Autodesk Fusion 360 part; units mm, degrees
(part 5 of 14)
  line L2013 (32.35, 52.7992) -> (32.35, 53.4088)
  line L2014 (32.35, 51.5292) -> (32.35, 52.1388)
  line L2015 (32.983, 52.1388) -> (32.733, 52.1388)
  line L2016 (56.818, 14.4648) -> (56.818, 13.8552)
  line L2017 (33.366, 53.4088) -> (33.366, 52.7992)
  line L2018 (32.733, 52.7992) -> (32.983, 52.7992)
  line L2019 (57.9882, 55.626) -> (58.5978, 55.626)
  line L2020 (33.408, 52.134) -> (32.308, 52.134)
  line L2021 (33.366, 53.4088) -> (33.366, 52.7992)
  line L2022 (27.259, 50.123) -> (27.859, 50.123)
  line L2023 (27.8638, 50.165) -> (27.2542, 50.165)
  line L2024 (27.259, 51.223) -> (27.259, 50.123)
  line L2025 (32.308, 52.134) -> (32.308, 51.534)
  line L2026 (58.5978, 54.993) -> (58.5978, 55.243)
  line L2027 (21.209, 34.3408) -> (21.209, 33.7312)
  line L2028 (56.86, 14.46) -> (55.76, 14.46)
  line L2029 (34.76, 35.491) -> (34.76, 34.891)
  line L2030 (32.308, 53.404) -> (32.308, 52.804)
  line L2031 (27.2542, 50.548) -> (27.8638, 50.548)
  line L2032 (27.859, 50.123) -> (27.859, 51.223)
  line L2033 (32.308, 52.804) -> (33.408, 52.804)
  line L2034 (33.366, 52.1388) -> (33.366, 51.5292)
  line L2035 (20.826, 33.7312) -> (20.826, 34.3408)
  line L2036 (20.193, 34.3408) -> (21.209, 34.3408)
  line L2037 (27.8638, 51.181) -> (27.8638, 50.165)
  line L2038 (32.35, 52.7992) -> (32.35, 53.4088)
  line L2039 (20.193, 34.3408) -> (21.209, 34.3408)
  line L2040 (27.2542, 50.165) -> (27.2542, 51.181)
  line L2041 (33.408, 51.534) -> (33.408, 52.134)
  line L2042 (27.8638, 51.181) -> (27.8638, 50.165)
  line L2043 (55.76, 14.46) -> (55.76, 13.86)
  line L2044 (56.435, 14.4648) -> (56.185, 14.4648)
  line L2045 (40.5638, 44.958) -> (40.5638, 43.942)
  line L2046 (39.9542, 44.958) -> (40.5638, 44.958)
  line L2047 (35.435, 36.7658) -> (35.185, 36.7658)
  line L2048 (34.802, 34.8862) -> (34.802, 35.4958)
  line L2049 (41.7068, 44.958) -> (41.7068, 43.942)
  line L2050 (35.818, 36.7658) -> (35.818, 36.1562)
  line L2051 (57.9882, 54.61) -> (57.9882, 55.626)
  line L2052 (35.818, 36.1562) -> (34.802, 36.1562)
  line L2053 (39.9542, 44.325) -> (40.5638, 44.325)
  line L2054 (39.9542, 44.958) -> (40.5638, 44.958)
  line L2055 (35.818, 35.4958) -> (35.818, 34.8862)
  line L2056 (41.102, 43.9) -> (41.702, 43.9)
  line L2057 (58.5978, 55.243) -> (57.9882, 55.243)
  line L2058 (35.185, 36.1562) -> (35.435, 36.1562)
  line L2059 (57.9882, 54.61) -> (57.9882, 55.626)
  line L2060 (27.8638, 50.548) -> (27.8638, 50.798)
  line L2061 (39.959, 45) -> (39.959, 43.9)
  line L2062 (35.185, 36.7658) -> (35.185, 36.1562)
  line L2063 (55.802, 14.4648) -> (56.818, 14.4648)
  line L2064 (34.802, 35.4958) -> (35.818, 35.4958)
  line L2065 (35.86, 35.491) -> (34.76, 35.491)
  line L2066 (58.5978, 55.626) -> (58.5978, 54.61)
  line L2067 (34.76, 34.891) -> (35.86, 34.891)
  line L2068 (27.2542, 50.798) -> (27.2542, 50.548)
  line L2069 (35.435, 35.4958) -> (35.185, 35.4958)
  line L2070 (39.9542, 43.942) -> (39.9542, 44.958)
  line L2071 (56.818, 13.8552) -> (55.802, 13.8552)
  line L2072 (41.0972, 44.958) -> (41.7068, 44.958)
  line L2073 (41.702, 43.9) -> (41.702, 45)
  line L2074 (55.76, 13.86) -> (56.86, 13.86)
  line L2075 (35.185, 35.4958) -> (35.185, 34.8862)
  line L2076 (56.185, 14.4648) -> (56.185, 13.8552)
  line L2077 (27.2542, 50.165) -> (27.2542, 51.181)
  line L2078 (35.86, 36.761) -> (34.76, 36.761)
  line L2079 (34.802, 35.4958) -> (35.818, 35.4958)
  line L2080 (41.7068, 43.942) -> (41.0972, 43.942)
  line L2081 (35.86, 36.161) -> (35.86, 36.761)
  line L2082 (56.435, 13.8552) -> (56.435, 14.4648)
  line L2083 (57.9882, 54.993) -> (58.5978, 54.993)
  line L2084 (41.7068, 43.942) -> (41.0972, 43.942)
  line L2085 (41.702, 45) -> (41.102, 45)
  line L2086 (55.802, 14.4648) -> (56.818, 14.4648)
  line L2087 (58.593, 55.668) -> (57.993, 55.668)
  line L2088 (41.0972, 44.325) -> (41.7068, 44.325)
  line L2089 (35.185, 34.8862) -> (35.435, 34.8862)
  line L2090 (39.959, 43.9) -> (40.559, 43.9)
  line L2091 (39.9542, 43.942) -> (39.9542, 44.958)
  line L2092 (55.802, 13.8552) -> (55.802, 14.4648)
  line L2093 (40.5638, 43.942) -> (39.9542, 43.942)
  line L2094 (58.593, 54.568) -> (58.593, 55.668)
  line L2095 (34.802, 34.8862) -> (34.802, 35.4958)
  line L2096 (58.5978, 54.61) -> (57.9882, 54.61)
  line L2097 (40.5638, 44.958) -> (40.5638, 43.942)
  line L2098 (57.9882, 55.243) -> (57.9882, 54.993)
  line L2099 (27.8638, 50.165) -> (27.2542, 50.165)
  line L2100 (34.802, 36.7658) -> (35.818, 36.7658)
  line L2101 (35.818, 34.8862) -> (34.802, 34.8862)
  line L2102 (35.86, 34.891) -> (35.86, 35.491)
  line L2103 (27.8638, 50.798) -> (27.2542, 50.798)
  line L2104 (40.5638, 43.942) -> (39.9542, 43.942)
  line L2105 (34.76, 36.161) -> (35.86, 36.161)
  line L2106 (41.7068, 44.575) -> (41.0972, 44.575)
  line L2107 (57.993, 55.668) -> (57.993, 54.568)
  line L2108 (41.0972, 43.942) -> (41.0972, 44.958)
  line L2109 (34.802, 31.3302) -> (34.802, 31.9398)
  line L2110 (35.185, 31.3302) -> (35.435, 31.3302)
  line L2111 (41.0972, 44.575) -> (41.0972, 44.325)
  line L2112 (35.435, 31.3302) -> (35.435, 31.9398)
  line L2113 (35.86, 31.935) -> (34.76, 31.935)
  line L2114 (37.6682, 43.942) -> (37.6682, 44.958)
  line L2115 (34.802, 31.9398) -> (35.818, 31.9398)
  line L2116 (38.816, 45) -> (38.816, 43.9)
  line L2117 (35.818, 31.9398) -> (35.818, 31.3302)
  line L2118 (34.802, 36.1562) -> (34.802, 36.7658)
  line L2119 (38.2778, 44.575) -> (37.6682, 44.575)
  line L2120 (41.102, 45) -> (41.102, 43.9)
  line L2121 (34.76, 31.935) -> (34.76, 31.335)
  line L2122 (39.4208, 43.942) -> (38.8112, 43.942)
  line L2123 (38.273, 45) -> (37.673, 45)
  line L2124 (38.2778, 43.942) -> (37.6682, 43.942)
  line L2125 (39.4208, 44.958) -> (39.4208, 43.942)
  line L2126 (37.673, 43.9) -> (38.273, 43.9)
  line L2127 (38.816, 43.9) -> (39.416, 43.9)
  line L2128 (38.8112, 43.942) -> (38.8112, 44.958)
  line L2129 (34.76, 36.761) -> (34.76, 36.161)
  line L2130 (38.2778, 44.958) -> (38.2778, 43.942)
  line L2131 (38.8112, 43.942) -> (38.8112, 44.958)
  line L2132 (41.7068, 44.958) -> (41.7068, 43.942)
  line L2133 (39.416, 43.9) -> (39.416, 45)
  line L2134 (35.818, 31.9398) -> (35.818, 31.3302)
  line L2135 (35.435, 31.9398) -> (35.185, 31.9398)
  line L2136 (37.6682, 44.958) -> (38.2778, 44.958)
  line L2137 (38.2778, 43.942) -> (37.6682, 43.942)
  line L2138 (38.273, 43.9) -> (38.273, 45)
  line L2139 (35.86, 31.335) -> (35.86, 31.935)
  line L2140 (35.185, 31.9398) -> (35.185, 31.3302)
  line L2141 (38.2778, 44.325) -> (38.2778, 44.575)
  line L2142 (38.2778, 44.958) -> (38.2778, 43.942)
  line L2143 (34.802, 31.3302) -> (34.802, 31.9398)
  line L2144 (35.818, 31.3302) -> (34.802, 31.3302)
  line L2145 (39.4208, 44.575) -> (38.8112, 44.575)
  line L2146 (39.4208, 44.325) -> (39.4208, 44.575)
  line L2147 (35.818, 36.7658) -> (35.818, 36.1562)
  line L2148 (37.6682, 44.325) -> (38.2778, 44.325)
  line L2149 (35.435, 36.1562) -> (35.435, 36.7658)
  line L2150 (37.6682, 44.958) -> (38.2778, 44.958)
  line L2151 (40.5638, 44.325) -> (40.5638, 44.575)
  line L2152 (38.8112, 44.958) -> (39.4208, 44.958)
  line L2153 (41.0972, 44.958) -> (41.7068, 44.958)
  line L2154 (37.6682, 44.575) -> (37.6682, 44.325)
  line L2155 (40.5638, 44.575) -> (39.9542, 44.575)
  line L2156 (40.559, 43.9) -> (40.559, 45)
  line L2157 (39.4208, 44.958) -> (39.4208, 43.942)
  line L2158 (38.8112, 44.575) -> (38.8112, 44.325)
  line L2159 (34.76, 31.335) -> (35.86, 31.335)
  line L2160 (40.559, 45) -> (39.959, 45)
  line L2161 (37.673, 45) -> (37.673, 43.9)
  line L2162 (34.802, 36.7658) -> (35.818, 36.7658)
  line L2163 (41.0972, 43.942) -> (41.0972, 44.958)
  line L2164 (41.7068, 44.325) -> (41.7068, 44.575)
  line L2165 (39.9542, 44.575) -> (39.9542, 44.325)
  line L2166 (34.802, 36.1562) -> (34.802, 36.7658)
  line L2167 (37.6682, 43.942) -> (37.6682, 44.958)
  line L2168 (39.416, 45) -> (38.816, 45)
  line L2169 (35.818, 36.1562) -> (34.802, 36.1562)
  line L2170 (35.818, 31.3302) -> (34.802, 31.3302)
  line L2171 (38.8112, 44.958) -> (39.4208, 44.958)
  line L2172 (39.4208, 43.942) -> (38.8112, 43.942)
  line L2173 (34.802, 32.4732) -> (34.802, 33.0828)
  line L2174 (34.685, 28.162) -> (34.685, 27.562)
  line L2175 (35.36, 27.5572) -> (35.36, 28.1668)
  line L2176 (35.435, 33.0828) -> (35.185, 33.0828)
  line L2177 (35.818, 33.0828) -> (35.818, 32.4732)
  line L2178 (35.818, 32.4732) -> (34.802, 32.4732)
  line L2179 (36.5252, 44.325) -> (37.1348, 44.325)
  line L2180 (35.743, 27.5572) -> (34.727, 27.5572)
  line L2181 (37.1348, 44.958) -> (37.1348, 43.942)
  line L2182 (76.4032, 61.214) -> (76.4032, 62.23)
  line L2183 (35.818, 32.4732) -> (34.802, 32.4732)
  line L2184 (36.53, 43.9) -> (37.13, 43.9)
  line L2185 (37.13, 43.9) -> (37.13, 45)
  line L2186 (37.1348, 44.958) -> (37.1348, 43.942)
  line L2187 (34.802, 31.9398) -> (35.818, 31.9398)
  line L2188 (34.727, 27.5572) -> (34.727, 28.1668)
  line L2189 (34.802, 33.0828) -> (35.818, 33.0828)
  line L2190 (35.743, 30.4528) -> (35.743, 29.8432)
  line L2191 (35.785, 28.705) -> (35.785, 29.305)
  line L2192 (36.5252, 44.958) -> (37.1348, 44.958)
  line L2193 (34.76, 33.078) -> (34.76, 32.478)
  line L2194 (35.743, 28.1668) -> (35.743, 27.5572)
  line L2195 (35.818, 33.0828) -> (35.818, 32.4732)
  line L2196 (35.785, 29.305) -> (34.685, 29.305)
  line L2197 (35.185, 33.0828) -> (35.185, 32.4732)
  line L2198 (35.11, 27.5572) -> (35.36, 27.5572)
  line L2199 (34.727, 28.7002) -> (34.727, 29.3098)
  line L2200 (34.802, 32.4732) -> (34.802, 33.0828)
  line L2201 (35.11, 30.4528) -> (35.11, 29.8432)
  line L2202 (35.743, 28.7002) -> (34.727, 28.7002)
  line L2203 (35.86, 32.478) -> (35.86, 33.078)
  line L2204 (35.743, 28.7002) -> (34.727, 28.7002)
  line L2205 (35.36, 28.1668) -> (35.11, 28.1668)
  line L2206 (34.727, 29.3098) -> (35.743, 29.3098)
  line L2207 (34.727, 28.7002) -> (34.727, 29.3098)
  line L2208 (35.785, 29.848) -> (35.785, 30.448)
  line L2209 (76.408, 62.272) -> (76.408, 61.172)
  line L2210 (34.685, 27.562) -> (35.785, 27.562)
  line L2211 (35.185, 32.4732) -> (35.435, 32.4732)
  line L2212 (35.11, 29.8432) -> (35.36, 29.8432)
  line L2213 (36.53, 45) -> (36.53, 43.9)
  line L2214 (35.36, 29.3098) -> (35.11, 29.3098)
  line L2215 (34.727, 28.1668) -> (35.743, 28.1668)
  line L2216 (35.11, 29.3098) -> (35.11, 28.7002)
  line L2217 (35.11, 28.1668) -> (35.11, 27.5572)
  line L2218 (34.685, 28.705) -> (35.785, 28.705)
  line L2219 (34.685, 29.305) -> (34.685, 28.705)
  line L2220 (35.785, 27.562) -> (35.785, 28.162)
  line L2221 (34.727, 28.1668) -> (35.743, 28.1668)
  line L2222 (34.727, 29.3098) -> (35.743, 29.3098)
  line L2223 (34.76, 32.478) -> (35.86, 32.478)
  line L2224 (35.435, 32.4732) -> (35.435, 33.0828)
  line L2225 (35.36, 28.7002) -> (35.36, 29.3098)
  line L2226 (38.8112, 44.325) -> (39.4208, 44.325)
  line L2227 (34.727, 27.5572) -> (34.727, 28.1668)
  line L2228 (35.743, 29.3098) -> (35.743, 28.7002)
  line L2229 (35.743, 28.1668) -> (35.743, 27.5572)
  line L2230 (35.86, 33.078) -> (34.76, 33.078)
  line L2231 (35.743, 27.5572) -> (34.727, 27.5572)
  line L2232 (34.802, 33.0828) -> (35.818, 33.0828)
  line L2233 (37.13, 45) -> (36.53, 45)
  line L2234 (35.785, 28.162) -> (34.685, 28.162)
  line L2235 (35.11, 28.7002) -> (35.36, 28.7002)
  line L2236 (35.743, 29.3098) -> (35.743, 28.7002)
  line L2237 (51.6128, 43.688) -> (51.0032, 43.688)
  line L2238 (37.1348, 43.942) -> (36.5252, 43.942)
  line L2239 (52.7304, 58.6438) -> (52.4764, 58.1358)
  line L2240 (51.608, 43.646) -> (51.608, 44.746)
  line L2241 (51.0032, 43.688) -> (51.0032, 44.704)
  line L2242 (51.0032, 44.704) -> (51.6128, 44.704)
  line L2243 (35.743, 29.8432) -> (34.727, 29.8432)
  line L2244 (55.4736, 60.9092) -> (54.5084, 60.9092)
  line L2245 (54.5084, 60.9092) -> (54.5084, 59.2328)
  line L2246 (55.4736, 59.2328) -> (55.4736, 60.9092)
  line L2247 (37.1348, 43.942) -> (36.5252, 43.942)
  line L2248 (52.9336, 59.2328) -> (52.9336, 60.9092)
  line L2249 (54.5084, 60.9092) -> (54.5084, 59.2328)
  line L2250 (51.6128, 44.071) -> (51.6128, 44.321)
  line L2251 (35.743, 30.4528) -> (35.743, 29.8432)
  line L2252 (36.5252, 44.958) -> (37.1348, 44.958)
  line L2253 (77.0128, 61.214) -> (76.4032, 61.214)
  line L2254 (77.008, 62.272) -> (76.408, 62.272)
  line L2255 (54.511, 60.946) -> (54.511, 59.196)
  line L2256 (52.4764, 58.1358) -> (52.2224, 58.6438)
  line L2257 (36.5252, 43.942) -> (36.5252, 44.958)
  line L2258 (34.727, 30.4528) -> (35.743, 30.4528)
  line L2259 (52.901, 60.771) -> (52.001, 60.771)
  line L2260 (52.2224, 58.6438) -> (52.7304, 58.6438)
  line L2261 (51.9684, 60.9092) -> (51.9684, 59.2328)
  line L2262 (52.9336, 60.9092) -> (51.9684, 60.9092)
  line L2263 (55.4736, 59.2328) -> (55.4736, 60.9092)
  line L2264 (54.5084, 59.2328) -> (55.4736, 59.2328)
  arc A1277 (52.2224, 58.085) -> (52.2224, 58.1866) centre (52.2224, 58.1358) ccw
  line L2265 (35.785, 30.448) -> (34.685, 30.448)
  arc A1278 (52.4764, 58.1866) -> (52.4764, 58.085) centre (52.4764, 58.1358) ccw
  line L2266 (51.008, 44.746) -> (51.008, 43.646)
  line L2267 (77.0128, 62.23) -> (77.0128, 61.214)
  line L2268 (34.685, 29.848) -> (35.785, 29.848)
  line L2269 (34.727, 29.8432) -> (34.727, 30.4528)
  line L2270 (37.1348, 44.575) -> (36.5252, 44.575)
  line L2271 (76.4032, 61.847) -> (76.4032, 61.597)
  line L2272 (51.0032, 43.688) -> (51.0032, 44.704)
  line L2273 (51.6128, 43.688) -> (51.0032, 43.688)
  line L2274 (76.4032, 62.23) -> (77.0128, 62.23)
  line L2275 (77.0128, 61.597) -> (77.0128, 61.847)
  line L2276 (51.6128, 44.704) -> (51.6128, 43.688)
  line L2277 (52.9336, 60.9092) -> (51.9684, 60.9092)
  line L2278 (77.0128, 61.847) -> (76.4032, 61.847)
  line L2279 (34.727, 30.4528) -> (35.743, 30.4528)
  line L2280 (35.36, 30.4528) -> (35.11, 30.4528)
  line L2281 (51.008, 43.646) -> (51.608, 43.646)
  line L2282 (77.008, 61.172) -> (77.008, 62.272)
  line L2283 (77.0128, 61.214) -> (76.4032, 61.214)
  line L2284 (51.608, 44.746) -> (51.008, 44.746)
  line L2285 (34.685, 30.448) -> (34.685, 29.848)
  line L2286 (51.6128, 44.321) -> (51.0032, 44.321)
  line L2287 (76.408, 61.172) -> (77.008, 61.172)
  line L2288 (36.5252, 44.575) -> (36.5252, 44.325)
  line L2289 (36.5252, 43.942) -> (36.5252, 44.958)
  line L2290 (35.36, 29.8432) -> (35.36, 30.4528)
  line L2291 (76.4032, 62.23) -> (77.0128, 62.23)
  line L2292 (37.1348, 44.325) -> (37.1348, 44.575)
  line L2293 (34.727, 29.8432) -> (34.727, 30.4528)
  line L2294 (35.743, 29.8432) -> (34.727, 29.8432)
  line L2295 (76.4032, 61.214) -> (76.4032, 62.23)
  line L2296 (54.5084, 59.2328) -> (55.4736, 59.2328)
  line L2297 (77.0128, 62.23) -> (77.0128, 61.214)
  line L2298 (76.4032, 61.597) -> (77.0128, 61.597)
  line L2299 (58.0136, 59.2328) -> (58.0136, 60.9092)
  arc A1279 (54.7624, 58.6946) -> (54.7624, 58.593) centre (54.7624, 58.6438) ccw
  line L2300 (52.9336, 59.2328) -> (52.9336, 60.9092)
  arc A1280 (57.3024, 58.085) -> (57.3024, 58.1866) centre (57.3024, 58.1358) ccw
  line L2301 (57.981, 60.771) -> (57.081, 60.771)
  arc A1281 (57.3024, 58.593) -> (57.3024, 58.6946) centre (57.3024, 58.6438) ccw
  arc A1282 (54.7624, 58.593) -> (54.7624, 58.6946) centre (54.7624, 58.6438) ccw
  line L2302 (51.971, 60.946) -> (51.971, 59.196)
  line L2303 (57.981, 60.771) -> (57.081, 60.771)
  line L2304 (52.931, 60.946) -> (51.971, 60.946)
  line L2305 (58.0136, 60.9092) -> (57.0484, 60.9092)
  line L2306 (51.0032, 44.704) -> (51.6128, 44.704)
  arc A1283 (52.7304, 58.1866) -> (52.7304, 58.085) centre (52.7304, 58.1358) ccw
  arc A1284 (57.8104, 58.593) -> (57.8104, 58.6946) centre (57.8104, 58.6438) ccw
  line L2307 (57.8104, 58.6438) -> (57.5564, 58.1358)
  line L2308 (58.0136, 60.9092) -> (57.0484, 60.9092)
  line L2309 (51.0032, 44.321) -> (51.0032, 44.071)
  arc A1285 (55.2704, 58.1866) -> (55.2704, 58.085) centre (55.2704, 58.1358) ccw
  line L2310 (58.011, 59.196) -> (58.011, 60.946)
  line L2311 (51.9684, 59.2328) -> (52.9336, 59.2328)
  arc A1286 (52.7304, 58.085) -> (52.7304, 58.1866) centre (52.7304, 58.1358) ccw
  line L2312 (52.7304, 58.1358) -> (52.2224, 58.1358)
  arc A1287 (55.2704, 58.6946) -> (55.2704, 58.593) centre (55.2704, 58.6438) ccw
  arc A1288 (52.2224, 58.6946) -> (52.2224, 58.593) centre (52.2224, 58.6438) ccw
  line L2313 (57.5564, 58.1358) -> (57.3024, 58.6438)
  arc A1289 (55.2704, 58.593) -> (55.2704, 58.6946) centre (55.2704, 58.6438) ccw
  arc A1290 (55.0164, 58.085) -> (55.0164, 58.1866) centre (55.0164, 58.1358) ccw
  arc A1291 (55.0164, 58.1866) -> (55.0164, 58.085) centre (55.0164, 58.1358) ccw
  arc A1292 (57.5564, 58.085) -> (57.5564, 58.1866) centre (57.5564, 58.1358) ccw
  arc A1293 (57.3024, 58.6946) -> (57.3024, 58.593) centre (57.3024, 58.6438) ccw
  line L2314 (55.441, 60.771) -> (54.541, 60.771)
  arc A1294 (57.3024, 58.1866) -> (57.3024, 58.085) centre (57.3024, 58.1358) ccw
  arc A1295 (52.4764, 58.085) -> (52.4764, 58.1866) centre (52.4764, 58.1358) ccw
  line L2315 (57.3024, 58.6438) -> (57.8104, 58.6438)
  line L2316 (57.051, 60.946) -> (57.051, 59.196)
  arc A1296 (57.5564, 58.1866) -> (57.5564, 58.085) centre (57.5564, 58.1358) ccw
  arc A1297 (57.8104, 58.1866) -> (57.8104, 58.085) centre (57.8104, 58.1358) ccw
  arc A1298 (52.2224, 58.1866) -> (52.2224, 58.085) centre (52.2224, 58.1358) ccw
  line L2317 (54.511, 59.196) -> (55.471, 59.196)
  line L2318 (57.0484, 60.9092) -> (57.0484, 59.2328)
  line L2319 (52.901, 59.371) -> (52.001, 59.371)
  arc A1299 (57.8104, 58.085) -> (57.8104, 58.1866) centre (57.8104, 58.1358) ccw
  line L2320 (52.931, 59.196) -> (52.931, 60.946)
  line L2321 (55.4736, 60.9092) -> (54.5084, 60.9092)
  line L2322 (52.901, 59.371) -> (52.001, 59.371)
  line L2323 (55.441, 59.371) -> (54.541, 59.371)
  line L2324 (51.0032, 44.071) -> (51.6128, 44.071)
  arc A1300 (52.2224, 58.593) -> (52.2224, 58.6946) centre (52.2224, 58.6438) ccw
  line L2325 (57.0484, 60.9092) -> (57.0484, 59.2328)
  arc A1301 (57.8104, 58.6946) -> (57.8104, 58.593) centre (57.8104, 58.6438) ccw
  arc A1302 (54.7624, 58.085) -> (54.7624, 58.1866) centre (54.7624, 58.1358) ccw
  line L2326 (52.901, 59.371) -> (52.001, 59.371)
  line L2327 (51.6128, 44.704) -> (51.6128, 43.688)
  line L2328 (55.471, 59.196) -> (55.471, 60.946)
  line L2329 (52.901, 60.771) -> (52.001, 60.771)
  line L2330 (51.9684, 59.2328) -> (52.9336, 59.2328)
  line L2331 (51.9684, 60.9092) -> (51.9684, 59.2328)
  arc A1303 (52.7304, 58.593) -> (52.7304, 58.6946) centre (52.7304, 58.6438) ccw
  arc A1304 (52.7304, 58.6946) -> (52.7304, 58.593) centre (52.7304, 58.6438) ccw
  line L2332 (55.471, 60.946) -> (54.511, 60.946)
  line L2333 (52.901, 60.771) -> (52.001, 60.771)
  line L2334 (51.971, 59.196) -> (52.931, 59.196)
  line L2335 (55.441, 60.771) -> (54.541, 60.771)
  line L2336 (58.0136, 59.2328) -> (58.0136, 60.9092)
  line L2337 (27.559, 10.5918) -> (27.559, 12.0142)
  line L2338 (25.566, 10.628) -> (25.566, 11.978)
  line L2339 (25.273, 12.0142) -> (25.273, 10.5918)
  line L2340 (15.41, 25.437) -> (17.61, 25.437)
  arc A1305 (55.2704, 58.085) -> (55.2704, 58.1866) centre (55.2704, 58.1358) ccw
  line L2341 (11.684, 23.3172) -> (11.684, 21.8948)
  line L2342 (28.575, 24.3078) -> (28.575, 25.7302)
  line L2343 (58.011, 60.946) -> (57.051, 60.946)
  line L2344 (57.8104, 58.1358) -> (57.3024, 58.1358)
  line L2345 (17.61, 26.887) -> (15.41, 26.887)
  line L2346 (13.97, 21.8948) -> (13.97, 23.3172)
  line L2347 (11.727, 23.331) -> (11.727, 21.881)
  line L2348 (27.266, 10.628) -> (27.266, 11.978)
  line L2349 (55.441, 59.371) -> (54.541, 59.371)
  line L2350 (13.97, 21.8948) -> (13.97, 23.3172)
  line L2351 (11.684, 21.8948) -> (13.97, 21.8948)
  line L2352 (55.0164, 58.1358) -> (54.7624, 58.6438)
  line L2353 (25.273, 12.0142) -> (25.273, 10.5918)
  line L2354 (25.316, 12.028) -> (25.316, 10.578)
  line L2355 (57.981, 59.371) -> (57.081, 59.371)
  line L2356 (11.977, 23.281) -> (11.977, 21.931)
  line L2357 (57.981, 59.371) -> (57.081, 59.371)
  line L2358 (27.516, 10.578) -> (27.516, 12.028)
  line L2359 (15.41, 26.887) -> (15.41, 25.437)
  line L2360 (15.367, 25.4508) -> (17.653, 25.4508)
  line L2361 (26.289, 25.7302) -> (26.289, 24.3078)
  line L2362 (11.684, 23.3172) -> (11.684, 21.8948)
  line L2363 (17.36, 26.837) -> (17.36, 25.487)
  line L2364 (13.677, 23.281) -> (13.677, 21.931)
  line L2365 (15.66, 26.837) -> (15.66, 25.487)
  line L2366 (57.0484, 59.2328) -> (58.0136, 59.2328)
  line L2367 (54.7624, 58.6438) -> (55.2704, 58.6438)
  line L2368 (55.441, 60.771) -> (54.541, 60.771)
  line L2369 (55.2704, 58.1358) -> (54.7624, 58.1358)
  line L2370 (25.566, 10.628) -> (25.566, 11.978)
  line L2371 (25.273, 10.5918) -> (27.559, 10.5918)
  line L2372 (13.927, 21.881) -> (13.927, 23.331)
  line L2373 (57.051, 59.196) -> (58.011, 59.196)
  line L2374 (57.981, 60.771) -> (57.081, 60.771)
  line L2375 (57.0484, 59.2328) -> (58.0136, 59.2328)
  line L2376 (13.97, 23.3172) -> (11.684, 23.3172)
  line L2377 (25.566, 10.628) -> (25.566, 11.978)
  line L2378 (11.727, 21.881) -> (13.927, 21.881)
  line L2379 (27.516, 12.028) -> (25.316, 12.028)
  line L2380 (13.677, 23.281) -> (13.677, 21.931)
  line L2381 (57.981, 59.371) -> (57.081, 59.371)
  line L2382 (27.559, 12.0142) -> (25.273, 12.0142)
  line L2383 (13.677, 23.281) -> (13.677, 21.931)
  arc A1306 (54.7624, 58.1866) -> (54.7624, 58.085) centre (54.7624, 58.1358) ccw
  line L2384 (11.977, 23.281) -> (11.977, 21.931)
  line L2385 (25.273, 10.5918) -> (27.559, 10.5918)
  line L2386 (55.2704, 58.6438) -> (55.0164, 58.1358)
  line L2387 (13.927, 23.331) -> (11.727, 23.331)
  line L2388 (28.575, 24.3078) -> (28.575, 25.7302)
  line L2389 (11.977, 23.281) -> (11.977, 21.931)
  line L2390 (28.282, 24.344) -> (28.282, 25.694)
  line L2391 (27.559, 12.0142) -> (25.273, 12.0142)
  line L2392 (25.316, 10.578) -> (27.516, 10.578)
  line L2393 (55.441, 59.371) -> (54.541, 59.371)
  line L2394 (27.559, 10.5918) -> (27.559, 12.0142)
  line L2395 (27.266, 10.628) -> (27.266, 11.978)
  line L2396 (27.266, 10.628) -> (27.266, 11.978)
  line L2397 (11.684, 21.8948) -> (13.97, 21.8948)
  line L2398 (13.97, 23.3172) -> (11.684, 23.3172)
  line L2399 (85.9028, 46.355) -> (87.3252, 46.355)
  line L2400 (94.1578, 21.971) -> (95.5802, 21.971)
  line L2401 (28.282, 24.344) -> (28.282, 25.694)
  line L2402 (94.1578, 24.257) -> (94.1578, 21.971)
  line L2403 (83.9978, 48.514) -> (83.9978, 46.228)
  line L2404 (85.939, 46.648) -> (87.289, 46.648)
  line L2405 (85.434, 46.271) -> (85.434, 48.471)
  line L2406 (85.434, 48.471) -> (83.984, 48.471)
  line L2407 (15.367, 26.8732) -> (15.367, 25.4508)
  line L2408 (94.144, 24.214) -> (94.144, 22.014)
  line L2409 (84.034, 46.521) -> (85.384, 46.521)
  line L2410 (17.36, 26.837) -> (17.36, 25.487)
  line L2411 (84.034, 46.521) -> (85.384, 46.521)
  line L2412 (26.582, 24.344) -> (26.582, 25.694)
  line L2413 (17.653, 25.4508) -> (17.653, 26.8732)
  line L2414 (28.575, 25.7302) -> (26.289, 25.7302)
  line L2415 (26.289, 24.3078) -> (28.575, 24.3078)
  line L2416 (85.9028, 48.641) -> (85.9028, 46.355)
  line L2417 (17.653, 26.8732) -> (15.367, 26.8732)
  line L2418 (26.332, 25.744) -> (26.332, 24.294)
  line L2419 (87.3252, 48.641) -> (85.9028, 48.641)
  line L2420 (17.61, 25.437) -> (17.61, 26.887)
  line L2421 (17.653, 26.8732) -> (15.367, 26.8732)
  line L2422 (87.339, 48.598) -> (85.889, 48.598)
  line L2423 (85.4202, 48.514) -> (83.9978, 48.514)
  line L2424 (26.332, 24.294) -> (28.532, 24.294)
  line L2425 (84.034, 48.221) -> (85.384, 48.221)
  line L2426 (94.1578, 21.971) -> (95.5802, 21.971)
  line L2427 (15.66, 26.837) -> (15.66, 25.487)
  line L2428 (85.939, 48.348) -> (87.289, 48.348)
  line L2429 (15.66, 26.837) -> (15.66, 25.487)
  line L2430 (83.9978, 48.514) -> (83.9978, 46.228)
  line L2431 (85.9028, 46.355) -> (87.3252, 46.355)
  line L2432 (83.9978, 46.228) -> (85.4202, 46.228)
  line L2433 (26.582, 24.344) -> (26.582, 25.694)
  line L2434 (26.582, 24.344) -> (26.582, 25.694)
  line L2435 (15.367, 25.4508) -> (17.653, 25.4508)
  line L2436 (26.289, 25.7302) -> (26.289, 24.3078)
  line L2437 (15.367, 26.8732) -> (15.367, 25.4508)
  line L2438 (28.575, 25.7302) -> (26.289, 25.7302)
  line L2439 (85.889, 48.598) -> (85.889, 46.398)
  line L2440 (26.289, 24.3078) -> (28.575, 24.3078)
  line L2441 (87.3252, 46.355) -> (87.3252, 48.641)
  line L2442 (17.653, 25.4508) -> (17.653, 26.8732)
  line L2443 (17.36, 26.837) -> (17.36, 25.487)
  line L2444 (28.282, 24.344) -> (28.282, 25.694)
  line L2445 (28.532, 25.744) -> (26.332, 25.744)
  line L2446 (85.4202, 48.514) -> (83.9978, 48.514)
  line L2447 (85.9028, 48.641) -> (85.9028, 46.355)
  line L2448 (85.939, 46.648) -> (87.289, 46.648)
  line L2449 (28.532, 24.294) -> (28.532, 25.744)
  line L2450 (87.339, 46.398) -> (87.339, 48.598)
  line L2451 (84.034, 48.221) -> (85.384, 48.221)
  line L2452 (95.594, 24.214) -> (94.144, 24.214)
  line L2453 (95.544, 22.264) -> (94.194, 22.264)
  line L2454 (87.3252, 48.641) -> (85.9028, 48.641)
  line L2455 (85.939, 48.348) -> (87.289, 48.348)
  line L2456 (85.4202, 46.228) -> (85.4202, 48.514)
  line L2457 (95.5802, 24.257) -> (94.1578, 24.257)
  line L2458 (85.939, 46.648) -> (87.289, 46.648)
  line L2459 (84.034, 48.221) -> (85.384, 48.221)
  line L2460 (84.034, 46.521) -> (85.384, 46.521)
  line L2461 (85.889, 46.398) -> (87.339, 46.398)
  line L2462 (94.144, 22.014) -> (95.594, 22.014)
  line L2463 (94.194, 40.474) -> (95.544, 40.474)
  line L2464 (83.9978, 46.228) -> (85.4202, 46.228)
  line L2465 (94.1578, 40.767) -> (94.1578, 38.481)
  line L2466 (94.1578, 54.229) -> (94.1578, 51.943)
  line L2467 (94.194, 38.774) -> (95.544, 38.774)
  line L2468 (94.1578, 51.943) -> (95.5802, 51.943)
  line L2469 (101.6, 33.909) -> (103.251, 33.909)
  line L2470 (95.5802, 38.481) -> (95.5802, 40.767)
  line L2471 (95.671, 7.278) -> (94.321, 7.278)
  line L2472 (95.544, 53.936) -> (94.194, 53.936)
  line L2473 (95.5802, 54.229) -> (94.1578, 54.229)
  line L2474 (95.544, 23.964) -> (94.194, 23.964)
  line L2475 (95.5802, 40.767) -> (94.1578, 40.767)
  line L2476 (94.2848, 6.985) -> (95.7072, 6.985)
  line L2477 (94.2848, 9.271) -> (94.2848, 6.985)
  line L2478 (95.671, 8.978) -> (94.321, 8.978)
  line L2479 (95.544, 22.264) -> (94.194, 22.264)
  line L2480 (95.721, 7.028) -> (95.721, 9.228)
  line L2481 (14.3002, 14.986) -> (12.8778, 14.986)
  line L2482 (95.5802, 21.971) -> (95.5802, 24.257)
  line L2483 (94.1578, 38.481) -> (95.5802, 38.481)
  line L2484 (95.544, 52.236) -> (94.194, 52.236)
  line L2485 (12.8778, 12.7) -> (14.3002, 12.7)
  line L2486 (14.264, 12.993) -> (12.914, 12.993)
  line L2487 (14.264, 14.693) -> (12.914, 14.693)
  line L2488 (95.544, 53.936) -> (94.194, 53.936)
  line L2489 (95.594, 40.724) -> (94.144, 40.724)
  line L2490 (94.1578, 54.229) -> (94.1578, 51.943)
  line L2491 (94.1578, 51.943) -> (95.5802, 51.943)
  line L2492 (94.2848, 6.985) -> (95.7072, 6.985)
  line L2493 (95.544, 23.964) -> (94.194, 23.964)
  line L2494 (83.984, 46.271) -> (85.434, 46.271)
  line L2495 (95.7072, 9.271) -> (94.2848, 9.271)
  line L2496 (94.1578, 38.481) -> (95.5802, 38.481)
  line L2497 (94.144, 38.524) -> (95.594, 38.524)
  line L2498 (94.194, 38.774) -> (95.544, 38.774)
  line L2499 (95.671, 8.978) -> (94.321, 8.978)
  line L2500 (94.194, 38.774) -> (95.544, 38.774)
  line L2501 (95.5802, 21.971) -> (95.5802, 24.257)
  line L2502 (94.1578, 40.767) -> (94.1578, 38.481)
  line L2503 (85.939, 48.348) -> (87.289, 48.348)
  line L2504 (83.984, 48.471) -> (83.984, 46.271)
  line L2505 (94.194, 40.474) -> (95.544, 40.474)
  line L2506 (94.271, 7.028) -> (95.721, 7.028)
  line L2507 (95.544, 22.264) -> (94.194, 22.264)
  line L2508 (94.1578, 24.257) -> (94.1578, 21.971)
  line L2509 (94.271, 9.228) -> (94.271, 7.028)
  line L2510 (95.5802, 40.767) -> (94.1578, 40.767)
  line L2511 (94.2848, 9.271) -> (94.2848, 6.985)
  line L2512 (94.194, 40.474) -> (95.544, 40.474)
  line L2513 (94.144, 40.724) -> (94.144, 38.524)
  line L2514 (95.7072, 6.985) -> (95.7072, 9.271)
  line L2515 (95.544, 23.964) -> (94.194, 23.964)
  line L2516 (95.671, 7.278) -> (94.321, 7.278)
  line L2517 (95.7072, 9.271) -> (94.2848, 9.271)
  line L2518 (95.7072, 6.985) -> (95.7072, 9.271)
  line L2519 (85.4202, 46.228) -> (85.4202, 48.514)
  line L2520 (95.594, 22.014) -> (95.594, 24.214)
  line L2521 (95.721, 9.228) -> (94.271, 9.228)
  line L2522 (87.3252, 46.355) -> (87.3252, 48.641)
  line L2523 (95.5802, 24.257) -> (94.1578, 24.257)
  line L2524 (95.594, 38.524) -> (95.594, 40.724)
  line L2525 (95.5802, 38.481) -> (95.5802, 40.767)
  line L2526 (95.671, 7.278) -> (94.321, 7.278)
  line L2527 (103.251, 43.688) -> (96.774, 43.688)
  line L2528 (110.617, 35.179) -> (111.125, 35.687)
  line L2529 (96.774, 38.989) -> (101.6, 38.989)
  line L2530 (96.774, 38.481) -> (96.774, 38.989)
  line L2531 (105.156, 35.941) -> (105.918, 35.179)
  line L2532 (95.594, 51.986) -> (95.594, 54.186)
  line L2533 (101.6, 42.672) -> (101.6, 38.989)
  line L2534 (111.125, 41.783) -> (110.617, 42.291)
  line L2535 (101.6, 38.481) -> (101.6, 34.925)
  line L2536 (103.632, 35.941) -> (103.632, 41.529)
  line L2537 (95.5802, 51.943) -> (95.5802, 54.229)
  line L2538 (94.144, 54.186) -> (94.144, 51.986)
  line L2539 (14.264, 12.993) -> (12.914, 12.993)
  line L2540 (105.156, 35.941) -> (105.918, 35.179)
  line L2541 (103.632, 41.529) -> (103.251, 41.91)
  line L2542 (95.5802, 51.943) -> (95.5802, 54.229)
  line L2543 (12.864, 12.743) -> (14.314, 12.743)
  line L2544 (12.8778, 12.7) -> (14.3002, 12.7)
  line L2545 (12.8778, 14.986) -> (12.8778, 12.7)
  line L2546 (103.251, 33.909) -> (103.251, 43.688)
  line L2547 (14.3002, 12.7) -> (14.3002, 14.986)
  line L2548 (14.264, 14.693) -> (12.914, 14.693)
  line L2549 (14.314, 12.743) -> (14.314, 14.943)
  line L2550 (101.6, 33.909) -> (96.774, 33.909)
  line L2551 (105.918, 35.179) -> (110.617, 35.179)
  line L2552 (111.125, 35.687) -> (111.125, 41.783)
  line L2553 (95.544, 52.236) -> (94.194, 52.236)
  line L2554 (96.774, 43.688) -> (96.774, 42.672)
  line L2555 (12.864, 14.943) -> (12.864, 12.743)
  line L2556 (96.774, 42.672) -> (101.6, 42.672)
  line L2557 (101.6, 38.481) -> (96.774, 38.481)
  line L2558 (14.314, 14.943) -> (12.864, 14.943)
  line L2559 (14.3002, 14.986) -> (12.8778, 14.986)
  line L2560 (96.774, 38.481) -> (101.6, 38.481)
  line L2561 (105.156, 41.529) -> (103.632, 41.529)
  line L2562 (14.264, 14.693) -> (12.914, 14.693)
  line L2563 (103.632, 35.941) -> (105.156, 35.941)
  line L2564 (96.774, 38.989) -> (96.774, 38.481)
  line L2565 (105.918, 42.291) -> (105.156, 41.529)
  line L2566 (101.6, 43.688) -> (96.774, 43.688)
  line L2567 (110.617, 42.291) -> (105.918, 42.291)
  line L2568 (95.671, 8.978) -> (94.321, 8.978)
  line L2569 (111.125, 41.783) -> (110.617, 42.291)
  line L2570 (95.5802, 54.229) -> (94.1578, 54.229)
  line L2571 (103.251, 43.688) -> (101.6, 43.688)
  line L2572 (96.774, 43.688) -> (96.774, 42.672)
  line L2573 (12.8778, 14.986) -> (12.8778, 12.7)
  line L2574 (105.156, 35.941) -> (105.156, 41.529)
  line L2575 (101.6, 38.989) -> (96.774, 38.989)
  line L2576 (101.219, 34.3535) -> (96.139, 34.3535)
  line L2577 (105.918, 35.179) -> (105.918, 42.291)
  line L2578 (96.774, 33.909) -> (96.774, 34.925)
  line L2579 (95.544, 53.936) -> (94.194, 53.936)
  line L2580 (101.219, 34.3535) -> (96.139, 34.3535)
  line L2581 (101.6, 43.688) -> (101.6, 33.909)
  line L2582 (111.125, 35.687) -> (111.125, 41.783)
  line L2583 (95.594, 54.186) -> (94.144, 54.186)
  line L2584 (103.251, 41.91) -> (103.251, 43.688)
  line L2585 (96.774, 42.672) -> (101.6, 42.672)
  line L2586 (14.264, 12.993) -> (12.914, 12.993)
  line L2587 (96.774, 34.925) -> (101.6, 34.925)
  line L2588 (14.3002, 12.7) -> (14.3002, 14.986)
  line L2589 (95.544, 52.236) -> (94.194, 52.236)
  line L2590 (94.144, 51.986) -> (95.594, 51.986)
  line L2591 (103.632, 35.941) -> (105.156, 35.941)
  line L2592 (103.251, 35.56) -> (103.632, 35.941)
  line L2593 (103.251, 50.8) -> (103.632, 51.181)
  line L2594 (101.219, 43.1165) -> (96.139, 43.1165)
  line L2595 (105.918, 57.531) -> (105.156, 56.769)
  line L2596 (105.156, 51.181) -> (105.156, 56.769)
  line L2597 (105.918, 50.419) -> (105.918, 57.531)
  line L2598 (96.774, 58.928) -> (96.774, 57.912)
  line L2599 (105.156, 41.529) -> (103.632, 41.529)
  line L2600 (103.251, 49.149) -> (103.251, 58.928)
  line L2601 (101.219, 43.1165) -> (96.139, 43.1165)
  line L2602 (101.219, 38.735) -> (96.139, 38.735)
  line L2603 (105.156, 51.181) -> (105.918, 50.419)
  line L2604 (101.219, 38.735) -> (96.139, 38.735)
  line L2605 (103.632, 56.769) -> (103.251, 57.15)
  line L2606 (103.251, 50.8) -> (103.632, 51.181)
  line L2607 (101.219, 34.3535) -> (96.139, 34.3535)
  line L2608 (103.632, 51.181) -> (105.156, 51.181)
  line L2609 (101.219, 34.3535) -> (96.139, 34.3535)
  line L2610 (110.617, 57.531) -> (105.918, 57.531)
  line L2611 (105.918, 50.419) -> (110.617, 50.419)
  line L2612 (105.918, 42.291) -> (105.156, 41.529)
  line L2613 (101.219, 43.1165) -> (96.139, 43.1165)
  line L2614 (111.125, 57.023) -> (110.617, 57.531)
  line L2615 (105.918, 50.419) -> (110.617, 50.419)
  line L2616 (111.125, 50.927) -> (111.125, 57.023)
  line L2617 (105.156, 51.181) -> (105.918, 50.419)
  line L2618 (111.125, 57.023) -> (110.617, 57.531)
  line L2619 (101.6, 53.721) -> (96.774, 53.721)
  line L2620 (96.774, 53.721) -> (96.774, 54.229)
  line L2621 (103.632, 41.529) -> (103.251, 41.91)
  line L2622 (103.251, 35.56) -> (103.632, 35.941)
  line L2623 (103.251, 58.928) -> (101.6, 58.928)
  line L2624 (103.251, 49.149) -> (103.251, 50.8)
  line L2625 (101.6, 34.925) -> (96.774, 34.925)
  line L2626 (96.774, 54.229) -> (101.6, 54.229)
  line L2627 (96.774, 33.909) -> (103.251, 33.909)
  line L2628 (96.774, 50.165) -> (101.6, 50.165)
  line L2629 (101.6, 57.912) -> (101.6, 54.229)
  line L2630 (110.617, 50.419) -> (111.125, 50.927)
  line L2631 (103.632, 56.769) -> (103.251, 57.15)
  line L2632 (101.219, 34.3535) -> (96.139, 34.3535)
  line L2633 (101.219, 43.1165) -> (96.139, 43.1165)
  line L2634 (101.219, 38.735) -> (96.139, 38.735)
  line L2635 (103.251, 33.909) -> (103.251, 35.56)
  line L2636 (110.617, 50.419) -> (111.125, 50.927)
  line L2637 (103.632, 51.181) -> (105.156, 51.181)
  line L2638 (96.774, 57.912) -> (101.6, 57.912)
  line L2639 (101.6, 54.229) -> (96.774, 54.229)
  line L2640 (110.617, 35.179) -> (111.125, 35.687)
  line L2641 (111.125, 50.927) -> (111.125, 57.023)
  line L2642 (105.918, 35.179) -> (110.617, 35.179)
  line L2643 (96.774, 57.912) -> (101.6, 57.912)
  line L2644 (101.6, 58.928) -> (101.6, 49.149)
  line L2645 (96.774, 34.925) -> (96.774, 33.909)
  line L2646 (110.617, 42.291) -> (105.918, 42.291)
  line L2647 (101.6, 49.149) -> (103.251, 49.149)
  line L2648 (101.219, 43.1165) -> (96.139, 43.1165)
  line L2649 (103.251, 58.928) -> (96.774, 58.928)
  line L2650 (101.219, 43.1165) -> (96.139, 43.1165)
  line L2651 (105.918, 57.531) -> (105.156, 56.769)
  line L2652 (101.6, 49.149) -> (96.774, 49.149)
  line L2653 (96.774, 58.928) -> (96.774, 57.912)
  line L2654 (103.632, 51.181) -> (103.632, 56.769)
  line L2655 (101.219, 53.975) -> (96.139, 53.975)
  line L2656 (101.6, 23.876) -> (96.774, 23.876)
  line L2657 (101.219, 28.5115) -> (96.139, 28.5115)
  line L2658 (110.617, 20.574) -> (111.125, 21.082)
  line L2659 (101.6, 24.384) -> (96.774, 24.384)
  line L2660 (96.774, 29.083) -> (96.774, 28.067)
  line L2661 (101.219, 49.5935) -> (96.139, 49.5935)
  line L2662 (103.251, 29.083) -> (101.6, 29.083)
  line L2663 (96.774, 20.32) -> (96.774, 19.304)
  line L2664 (103.632, 26.924) -> (103.251, 27.305)
  line L2665 (96.774, 23.876) -> (96.774, 24.384)
  line L2666 (96.774, 24.384) -> (101.6, 24.384)
  line L2667 (96.774, 19.304) -> (96.774, 20.32)
  line L2668 (101.6, 19.304) -> (103.251, 19.304)
  line L2669 (96.774, 29.083) -> (96.774, 28.067)
  line L2670 (111.125, 27.178) -> (110.617, 27.686)
  line L2671 (101.6, 50.165) -> (96.774, 50.165)
  line L2672 (110.617, 20.574) -> (111.125, 21.082)
  line L2673 (96.774, 54.229) -> (96.774, 53.721)
  line L2674 (101.6, 19.304) -> (96.774, 19.304)
  line L2675 (105.918, 20.574) -> (105.918, 27.686)
  line L2676 (101.219, 53.975) -> (96.139, 53.975)
  line L2677 (103.632, 21.336) -> (105.156, 21.336)
  line L2678 (101.219, 49.5935) -> (96.139, 49.5935)
  line L2679 (101.6, 28.067) -> (101.6, 24.384)
  line L2680 (101.219, 28.5115) -> (96.139, 28.5115)
  line L2681 (101.219, 58.3565) -> (96.139, 58.3565)
  line L2682 (105.918, 20.574) -> (110.617, 20.574)
  line L2683 (103.251, 20.955) -> (103.632, 21.336)
  line L2684 (101.219, 24.13) -> (96.139, 24.13)
  line L2685 (105.156, 21.336) -> (105.156, 26.924)
  line L2686 (101.219, 58.3565) -> (96.139, 58.3565)
  line L2687 (101.219, 58.3565) -> (96.139, 58.3565)
  line L2688 (105.918, 27.686) -> (105.156, 26.924)
  line L2689 (103.251, 20.955) -> (103.632, 21.336)
  line L2690 (101.219, 49.5935) -> (96.139, 49.5935)
  line L2691 (96.774, 28.067) -> (101.6, 28.067)
  line L2692 (96.774, 20.32) -> (101.6, 20.32)
  line L2693 (103.251, 57.15) -> (103.251, 58.928)
  line L2694 (101.219, 58.3565) -> (96.139, 58.3565)
  line L2695 (101.219, 58.3565) -> (96.139, 58.3565)
  line L2696 (110.617, 57.531) -> (105.918, 57.531)
  line L2697 (105.156, 21.336) -> (105.918, 20.574)
  line L2698 (101.219, 53.975) -> (96.139, 53.975)
  line L2699 (96.774, 49.149) -> (96.774, 50.165)
  line L2700 (101.6, 58.928) -> (96.774, 58.928)
  line L2701 (101.219, 34.3535) -> (96.139, 34.3535)
  line L2702 (105.918, 20.574) -> (110.617, 20.574)
  line L2703 (101.219, 49.5935) -> (96.139, 49.5935)
  line L2704 (101.6, 53.721) -> (101.6, 50.165)
  line L2705 (105.156, 56.769) -> (103.632, 56.769)
  line L2706 (101.219, 49.5935) -> (96.139, 49.5935)
  line L2707 (101.6, 29.083) -> (101.6, 19.304)
  line L2708 (101.219, 49.5935) -> (96.139, 49.5935)
  line L2709 (96.774, 53.721) -> (101.6, 53.721)
  line L2710 (96.774, 49.149) -> (103.251, 49.149)
  line L2711 (110.617, 27.686) -> (105.918, 27.686)
  line L2712 (96.774, 50.165) -> (96.774, 49.149)
  line L2713 (103.251, 19.304) -> (103.251, 29.083)
  line L2714 (96.774, 28.067) -> (101.6, 28.067)
  line L2715 (105.156, 56.769) -> (103.632, 56.769)
  line L2716 (101.219, 58.3565) -> (96.139, 58.3565)
  line L2717 (101.6, 29.083) -> (96.774, 29.083)
  line L2718 (111.125, 21.082) -> (111.125, 27.178)
  line L2719 (103.251, 29.083) -> (96.774, 29.083)
  line L2720 (103.251, 19.304) -> (103.251, 20.955)
  line L2721 (96.774, 5.08) -> (96.774, 4.064)
  line L2722 (111.125, 27.178) -> (110.617, 27.686)
  line L2723 (105.918, 5.334) -> (110.617, 5.334)
  line L2724 (111.125, 21.082) -> (111.125, 27.178)
  line L2725 (105.918, 27.686) -> (105.156, 26.924)
  line L2726 (101.219, 19.7485) -> (96.139, 19.7485)
  line L2727 (105.918, 12.446) -> (105.156, 11.684)
  line L2728 (103.632, 11.684) -> (103.251, 12.065)
  line L2729 (105.156, 26.924) -> (103.632, 26.924)
  line L2730 (101.6, 5.08) -> (96.774, 5.08)
  line L2731 (96.774, 8.636) -> (96.774, 9.144)
  line L2732 (110.617, 5.334) -> (111.125, 5.842)
  line L2733 (101.219, 19.7485) -> (96.139, 19.7485)
  line L2734 (103.251, 4.064) -> (103.251, 13.843)
  line L2735 (105.156, 21.336) -> (105.918, 20.574)
  line L2736 (103.251, 5.715) -> (103.632, 6.096)
  line L2737 (96.774, 19.304) -> (103.251, 19.304)
  line L2738 (101.219, 24.13) -> (96.139, 24.13)
  line L2739 (110.617, 27.686) -> (105.918, 27.686)
  line L2740 (103.632, 21.336) -> (103.632, 26.924)
  line L2741 (103.251, 27.305) -> (103.251, 29.083)
  line L2742 (101.219, 28.5115) -> (96.139, 28.5115)
  line L2743 (96.774, 9.144) -> (101.6, 9.144)
  line L2744 (111.125, 11.938) -> (110.617, 12.446)
  line L2745 (96.774, 24.384) -> (96.774, 23.876)
  line L2746 (96.774, 5.08) -> (101.6, 5.08)
  line L2747 (103.251, 5.715) -> (103.632, 6.096)
  line L2748 (101.219, 19.7485) -> (96.139, 19.7485)
  line L2749 (101.6, 4.064) -> (103.251, 4.064)
  line L2750 (101.219, 28.5115) -> (96.139, 28.5115)
  line L2751 (103.251, 13.843) -> (101.6, 13.843)
  line L2752 (110.617, 12.446) -> (105.918, 12.446)
  line L2753 (105.156, 11.684) -> (103.632, 11.684)
  line L2754 (111.125, 5.842) -> (111.125, 11.938)
  line L2755 (111.125, 5.842) -> (111.125, 11.938)
  line L2756 (110.617, 12.446) -> (105.918, 12.446)
  line L2757 (101.6, 13.843) -> (101.6, 4.064)
  line L2758 (103.251, 4.064) -> (103.251, 5.715)
  line L2759 (101.219, 19.7485) -> (96.139, 19.7485)
  line L2760 (101.6, 20.32) -> (96.774, 20.32)
  line L2761 (101.219, 24.13) -> (96.139, 24.13)
  line L2762 (105.156, 6.096) -> (105.156, 11.684)
  line L2763 (103.632, 21.336) -> (105.156, 21.336)
  line L2764 (96.774, 12.827) -> (101.6, 12.827)
  line L2765 (96.774, 8.636) -> (101.6, 8.636)
  line L2766 (101.6, 23.876) -> (101.6, 20.32)
  line L2767 (103.632, 11.684) -> (103.251, 12.065)
  line L2768 (101.219, 4.5085) -> (96.139, 4.5085)
  line L2769 (103.632, 26.924) -> (103.251, 27.305)
  line L2770 (96.774, 13.843) -> (96.774, 12.827)
  line L2771 (101.219, 28.5115) -> (96.139, 28.5115)
  line L2772 (110.617, 5.334) -> (111.125, 5.842)
  line L2773 (101.219, 19.7485) -> (96.139, 19.7485)
  line L2774 (105.918, 5.334) -> (105.918, 12.446)
  line L2775 (96.774, 9.144) -> (96.774, 8.636)
  line L2776 (101.219, 19.7485) -> (96.139, 19.7485)
  line L2777 (105.156, 11.684) -> (103.632, 11.684)
  line L2778 (96.774, 23.876) -> (101.6, 23.876)
  line L2779 (105.156, 26.924) -> (103.632, 26.924)
  line L2780 (101.6, 13.843) -> (96.774, 13.843)
  line L2781 (101.6, 8.636) -> (101.6, 5.08)
  line L2782 (103.632, 6.096) -> (105.156, 6.096)
  line L2783 (101.219, 4.5085) -> (96.139, 4.5085)
  arc A1307 (3.81, 15.24) -> (3.81, 17.018) centre (3.81, 16.129) ccw
  line L2784 (101.219, 13.2715) -> (96.139, 13.2715)
  line L2785 (4.064, 16.129) -> (3.556, 16.129)
  arc A1308 (77.273, 24.8351) -> (77.273, 25.0129) centre (77.273, 24.924) ccw
  line L2786 (3.81, 15.875) -> (3.81, 16.383)
  line L2787 (101.219, 4.5085) -> (96.139, 4.5085)
  line L2788 (101.219, 13.2715) -> (96.139, 13.2715)
  line L2789 (3.81, 15.875) -> (3.81, 16.383)
  line L2790 (-3.81, 11.7094) -> (10.16, 11.7094)
  line L2791 (103.632, 6.096) -> (103.632, 11.684)
  arc A1309 (3.81, 17.018) -> (3.81, 15.24) centre (3.81, 16.129) ccw
  arc A1310 (3.81, 15.24) -> (3.81, 17.018) centre (3.81, 16.129) ccw
  arc A1311 (3.81, 15.24) -> (3.81, 17.018) centre (3.81, 16.129) ccw
  line L2792 (4.064, 16.129) -> (3.556, 16.129)
  line L2793 (101.6, 4.064) -> (96.774, 4.064)
  line L2794 (103.251, 12.065) -> (103.251, 13.843)
  line L2795 (4.064, 16.129) -> (3.556, 16.129)
  line L2796 (4.064, 16.129) -> (3.556, 16.129)
  line L2797 (101.219, 13.2715) -> (96.139, 13.2715)
  arc A1312 (3.81, 17.018) -> (3.81, 15.24) centre (3.81, 16.129) ccw
  line L2798 (105.918, 12.446) -> (105.156, 11.684)
  line L2799 (4.064, 16.129) -> (3.556, 16.129)
  arc A1313 (3.81, 17.018) -> (3.81, 15.24) centre (3.81, 16.129) ccw
  line L2800 (101.219, 8.89) -> (96.139, 8.89)
  line L2801 (101.219, 13.2715) -> (96.139, 13.2715)
  arc A1314 (3.81, 17.018) -> (3.81, 15.24) centre (3.81, 16.129) ccw
  arc A1315 (3.81, 15.24) -> (3.81, 17.018) centre (3.81, 16.129) ccw
  arc A1316 (3.81, 17.018) -> (3.81, 15.24) centre (3.81, 16.129) ccw
  arc A1317 (3.81, 17.018) -> (3.81, 15.24) centre (3.81, 16.129) ccw
  line L2802 (3.81, 15.875) -> (3.81, 16.383)
  line L2803 (101.219, 8.89) -> (96.139, 8.89)
  line L2804 (101.6, 9.144) -> (96.774, 9.144)
  line L2805 (10.16, 20.5994) -> (-3.81, 20.5994)
  line L2806 (3.81, 15.875) -> (3.81, 16.383)
  line L2807 (-3.81, 20.5994) -> (-3.81, 11.7094)
  arc A1318 (3.81, 15.24) -> (3.81, 17.018) centre (3.81, 16.129) ccw
  line L2808 (101.219, 13.2715) -> (96.139, 13.2715)
  line L2809 (3.81, 15.875) -> (3.81, 16.383)
  line L2810 (96.774, 4.064) -> (96.774, 5.08)
  line L2811 (101.219, 28.5115) -> (96.139, 28.5115)
  line L2812 (105.918, 5.334) -> (110.617, 5.334)
  line L2813 (103.632, 6.096) -> (105.156, 6.096)
  line L2814 (101.219, 4.5085) -> (96.139, 4.5085)
  line L2815 (105.156, 6.096) -> (105.918, 5.334)
  line L2816 (103.251, 13.843) -> (96.774, 13.843)
  line L2817 (96.774, 4.064) -> (103.251, 4.064)
  line L2818 (101.6, 12.827) -> (101.6, 9.144)
  line L2819 (4.064, 16.129) -> (3.556, 16.129)
  line L2820 (105.156, 6.096) -> (105.918, 5.334)
  arc A1319 (3.81, 15.24) -> (3.81, 17.018) centre (3.81, 16.129) ccw
  line L2821 (101.219, 4.5085) -> (96.139, 4.5085)
  line L2822 (96.774, 13.843) -> (96.774, 12.827)
  line L2823 (4.064, 16.129) -> (3.556, 16.129)
  line L2824 (3.81, 15.875) -> (3.81, 16.383)
  arc A1320 (3.81, 17.018) -> (3.81, 15.24) centre (3.81, 16.129) ccw
  line L2825 (111.125, 11.938) -> (110.617, 12.446)
  line L2826 (10.16, 11.7094) -> (10.16, 20.5994)
  line L2827 (3.81, 15.875) -> (3.81, 16.383)
  line L2828 (101.219, 13.2715) -> (96.139, 13.2715)
  line L2829 (101.219, 8.89) -> (96.139, 8.89)
  line L2830 (101.219, 4.5085) -> (96.139, 4.5085)
  line L2831 (101.6, 8.636) -> (96.774, 8.636)
  line L2832 (96.774, 12.827) -> (101.6, 12.827)
  line L2833 (5.6061, 14.3329) -> (5.6959, 14.2431)
  line L2834 (4.064, 16.129) -> (3.556, 16.129)
  arc A1321 (1.143, 16.129) -> (6.477, 16.129) centre (3.81, 16.129) ccw
  arc A1322 (2.54, 16.129) -> (5.08, 16.129) centre (3.81, 16.129) ccw
  arc A1323 (1.27, 16.129) -> (6.35, 16.129) centre (3.81, 16.129) ccw
  line L2835 (5.6061, 14.3329) -> (5.6959, 14.2431)
  arc A1324 (1.27, 16.129) -> (6.35, 16.129) centre (3.81, 16.129) ccw
  line L2836 (3.81, 15.875) -> (3.81, 16.383)
  line L2837 (2.0139, 14.3329) -> (1.9241, 14.2431)
  line L2838 (10.16, 15.875) -> (10.16, 16.383)
  arc A1325 (5.08, 16.129) -> (2.54, 16.129) centre (3.81, 16.129) ccw
  arc A1326 (3.81, 17.018) -> (3.81, 15.24) centre (3.81, 16.129) ccw
  arc A1327 (10.16, 16.9227) -> (10.16, 15.3352) centre (10.16, 16.129) ccw
  arc A1328 (2.54, 16.129) -> (5.08, 16.129) centre (3.81, 16.129) ccw
  arc A1329 (3.81, 15.24) -> (3.81, 17.018) centre (3.81, 16.129) ccw
  arc A1330 (5.08, 16.129) -> (2.54, 16.129) centre (3.81, 16.129) ccw
  arc A1331 (2.54, 16.129) -> (5.08, 16.129) centre (3.81, 16.129) ccw
  line L2839 (4.064, 16.129) -> (3.556, 16.129)
  arc A1332 (3.81, 15.24) -> (3.81, 17.018) centre (3.81, 16.129) ccw
  arc A1333 (3.81, 17.018) -> (3.81, 15.24) centre (3.81, 16.129) ccw
  line L2840 (10.414, 16.129) -> (9.906, 16.129)
  line L2841 (2.0139, 17.9251) -> (1.9241, 18.0149)
  line L2842 (5.6061, 17.9251) -> (5.6959, 18.0149)
  line L2843 (3.81, 15.875) -> (3.81, 16.383)
  line L2844 (5.6061, 17.9251) -> (5.6959, 18.0149)
  arc A1334 (1.27, 16.129) -> (6.35, 16.129) centre (3.81, 16.129) ccw
  arc A1335 (10.16, 15.3352) -> (10.16, 16.9227) centre (10.16, 16.129) ccw
  line L2845 (10.414, 16.129) -> (9.906, 16.129)
  line L2846 (4.064, 16.129) -> (3.556, 16.129)
  line L2847 (2.0139, 17.9251) -> (1.9241, 18.0149)
  arc A1336 (6.35, 16.129) -> (1.27, 16.129) centre (3.81, 16.129) ccw
  arc A1337 (1.143, 16.129) -> (6.477, 16.129) centre (3.81, 16.129) ccw
  arc A1338 (3.81, 15.24) -> (3.81, 17.018) centre (3.81, 16.129) ccw
  line L2848 (3.81, 15.875) -> (3.81, 16.383)
  arc A1339 (2.54, 16.129) -> (5.08, 16.129) centre (3.81, 16.129) ccw
  arc A1340 (10.16, 16.9227) -> (10.16, 15.3352) centre (10.16, 16.129) ccw
  line L2849 (2.0139, 14.3329) -> (1.9241, 14.2431)
  arc A1341 (6.477, 16.129) -> (1.143, 16.129) centre (3.81, 16.129) ccw
  line L2850 (5.6061, 14.3329) -> (5.6959, 14.2431)
  arc A1342 (6.35, 16.129) -> (1.27, 16.129) centre (3.81, 16.129) ccw
  line L2851 (2.0139, 14.3329) -> (1.9241, 14.2431)
  arc A1343 (10.16, 15.3352) -> (10.16, 16.9227) centre (10.16, 16.129) ccw
  arc A1344 (6.477, 16.129) -> (1.143, 16.129) centre (3.81, 16.129) ccw
  arc A1345 (5.08, 16.129) -> (2.54, 16.129) centre (3.81, 16.129) ccw
  line L2852 (10.16, 15.875) -> (10.16, 16.383)
  arc A1346 (3.81, 17.018) -> (3.81, 15.24) centre (3.81, 16.129) ccw
  arc A1347 (5.08, 16.129) -> (2.54, 16.129) centre (3.81, 16.129) ccw
  arc A1348 (5.08, 16.129) -> (2.54, 16.129) centre (3.81, 16.129) ccw
  line L2853 (2.0139, 17.9251) -> (1.9241, 18.0149)
  arc A1349 (10.16, 15.3352) -> (10.16, 16.9227) centre (10.16, 16.129) ccw
  line L2854 (10.414, 16.129) -> (9.906, 16.129)
  arc A1350 (2.54, 16.129) -> (5.08, 16.129) centre (3.81, 16.129) ccw
  arc A1351 (6.35, 16.129) -> (1.27, 16.129) centre (3.81, 16.129) ccw
  arc A1352 (1.143, 16.129) -> (6.477, 16.129) centre (3.81, 16.129) ccw
  arc A1353 (6.477, 16.129) -> (1.143, 16.129) centre (3.81, 16.129) ccw
  arc A1354 (3.81, 15.24) -> (3.81, 17.018) centre (3.81, 16.129) ccw
  arc A1355 (10.16, 16.9227) -> (10.16, 15.3352) centre (10.16, 16.129) ccw
  arc A1356 (82.693, 13.6558) -> (82.693, 13.5542) centre (82.693, 13.605) ccw
  arc A1357 (83.042, 40.7002) -> (83.042, 40.8018) centre (83.042, 40.751) ccw
  line L2855 (82.542, 40.5135) -> (82.542, 40.9885)
  line L2856 (81.2795, 39.251) -> (80.8045, 39.251)
  line L2857 (83.042, 40.751) -> (81.042, 40.751)
  line L2858 (83.2795, 39.251) -> (82.8045, 39.251)
  line L2859 (82.042, 40.5135) -> (82.042, 40.9885)
  line L2860 (75.3115, 40.124) -> (75.7865, 40.124)
  arc A1358 (81.042, 38.8018) -> (81.042, 38.7002) centre (81.042, 38.751) ccw
  line L2861 (83.193, 13.3675) -> (83.193, 13.8425)
  line L2862 (81.2795, 40.251) -> (80.8045, 40.251)
  line L2863 (81.542, 38.5135) -> (81.542, 38.9885)
  line L2864 (75.3115, 39.624) -> (75.7865, 39.624)
  line L2865 (81.042, 40.751) -> (81.042, 38.751)
  line L2866 (82.542, 40.5135) -> (82.542, 40.9885)
  line L2867 (82.042, 38.5135) -> (82.042, 38.9885)
  arc A1359 (81.042, 40.8018) -> (81.042, 40.7002) centre (81.042, 40.751) ccw
  arc A1360 (82.7386, 13.0751) -> (82.7386, 13.3061) centre (82.7386, 13.1906) ccw
  line L2868 (83.193, 13.3675) -> (83.193, 13.8425)
  line L2869 (83.2795, 39.751) -> (82.8045, 39.751)
  line L2870 (83.693, 13.3675) -> (83.693, 13.8425)